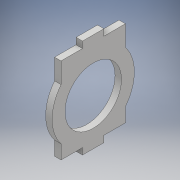
# Autodesk Inventor part: cod
Saved by Autodesk Inventor 2018 (Build 220112000, 112)
## iProperties
Created: 2020-03-11
Part Number: cod
Material: Genérico
Document SubType Name: Modeling
Designer: sala.ceri
Density: 1 g/cm^3
Appearance: Valor por defecto
Author: sala.ceri
Autodesk Inventor part; units mm, degrees
ref_plane "YZ Plane" through (0, 0, 0) normal (1, 0, 0) x (0, 1, 0)
ref_plane "XZ Plane" through (0, 0, 0) normal (0, 1, 0) x (-1, 0, 0)
ref_plane "XY Plane" through (0, 0, 0) normal (0, 0, 1) x (1, 0, 0)
sketch "Boceto1" plane through (0, 0, 0) normal (1, 0, 0) x (0, 1, 0)
  line L0 (0, 0) -> (0, -3)
  line L1 (0, -3) -> (10, -3)
  line L2 (10, -3) -> (10, 0)
  line L3 (10, 0) -> (20, 0)
  line L4 (20, 0) -> (20, -3)
  line L5 (20, -3) -> (30, -3)
  line L6 (30, -33.4269) -> (30, -40)
  line L7 (30, -40) -> (20, -40)
  line L8 (20, -40) -> (20, -43)
  line L9 (20, -43) -> (10, -43)
  line L10 (10, -43) -> (10, -40)
  line L11 (10, -40) -> (0, -40)
  circle A0 centre (15, -21.5) radius 13.175
  arc A1 (0, -9.5731) -> (0, -33.4269) centre (15, -21.5) ccw
  arc A2 (30, -33.4269) -> (30, -9.5731) centre (15, -21.5) ccw
  line L12 (0, -40) -> (0, -33.4269)
  line L13 (0, -9.5731) -> (0, -3)
  line L14 (30, -3) -> (30, -9.5731)
  dimension "d1" = 10
  dimension "d2" = 10
  dimension "d3" = 10
  constraints: 30 end point, 9 perpendicular, 9 point on line, 4 point on circle, 3 centre point, 2 parallel, 1 coincident, 1 vertical
  measures "d1" distance of L0.end L1.end
  measures "d2" distance of L2.end L3.end
  measures "d3" distance of L4.end L5.end
extrude "Extrusión1" add sketch "Boceto1" along normal blind 3
sketch "Boceto2" plane through (3, 0, 0) normal (1, 0, 0) x (0, 0, -1)
  line L0 (3, 10) -> (3, 0) projected
  line L1 (3, 0) -> (0, 0)
  line L2 (0, 20) -> (0, 10) projected
  line L3 (0, 0) -> (0, 10)
  line L4 (0, 10) -> (-3, 10)
  line L5 (-3, 10) -> (-3, 20)
  line L6 (-3, 20) -> (0, 20)
  line L7 (0, 20) -> (0, 30)
  line L8 (3, 30) -> (3, 20) projected
  line L9 (0, 30) -> (3, 30)
  line L10 (3, 30) -> (3, 20)
  line L11 (3, 20) -> (0, 20) projected
  line L12 (3, 20) -> (0, 20)
  line L13 (0, 20) -> (0, 10)
  line L14 (0, 10) -> (3, 10)
  line L15 (3, 0) -> (3, 10)
  dimension "d11" = 3
  constraints: 24 end point, 7 perpendicular, 3 point on line, 2 collinear, 1 horizontal
  measures "d11" distance of L2.end L4.end
extrude "Extrusión2" add sketch "Boceto2" against normal blind 3
